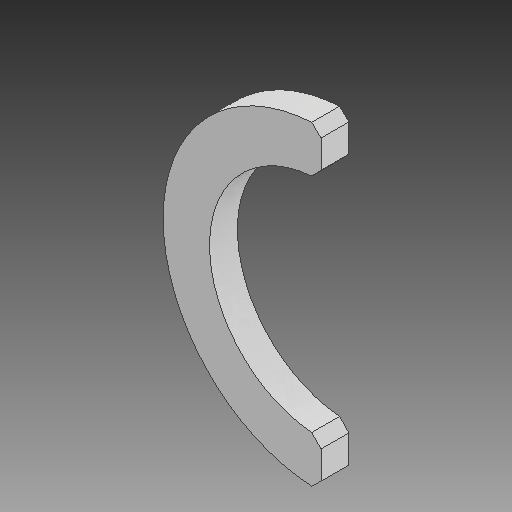
# Autodesk Inventor part: Ограничитель
Saved by Autodesk Inventor 2022 (Build 260153000, 153)
## iProperties
Created: 2025-01-25
Part Number: Ограничитель
Material: Типовые
Document SubType Name: Modeling
Designer: Ivan
Density: 1 g/cm^3
Appearance: По умолчанию
Author: Ivan
Autodesk Inventor part; units mm, degrees
ref_plane "YZ Plane" through (0, 0, 0) normal (1, 0, 0) x (0, 1, 0)
ref_plane "XZ Plane" through (0, 0, 0) normal (0, 1, 0) x (-1, 0, 0)
ref_plane "РабПлоскость1" through (0, 0, 6) normal (0, 0, 1) x (1, 0, 0)
sketch "Эскиз1" plane through (0, 0, 6) normal (0, 0, 1) x (1, 0, 0)
  circle A0 centre (36.1426, 85.1467) radius 24 projected
  circle A1 centre (36.1426, 85.1467) radius 34
  line L0 (36.1426, 85.1467) -> (36.1426, 122.276)
  line L1 (36.1426, 85.1467) -> (36.1426, 47.1457)
  point P0 (0, 0)
  point P1 (36.1426, 51.1467)
  point P2 (36.1426, 61.1467)
  point P3 (36.1426, 109.1467)
  point P4 (36.1426, 119.1467)
  dimension "d0" = 10
  constraints: 4 end point, 2 vertical, 1 centre point, 1 coincident
  measures "d0" radial gap between concentric circles of A0 A1
extrude "Выдавливание1" add sketch "Эскиз1" along normal blind 6 contours A0 L1 A1 L0 picked at (26.249, 113.9534)
chamfer "Фаска1" distance 2 angle 45 4 edges at (36.1426, 119.1467, 9) (36.1426, 109.1467, 9) (36.1426, 61.1467, 9) (36.1426, 51.1467, 9)
